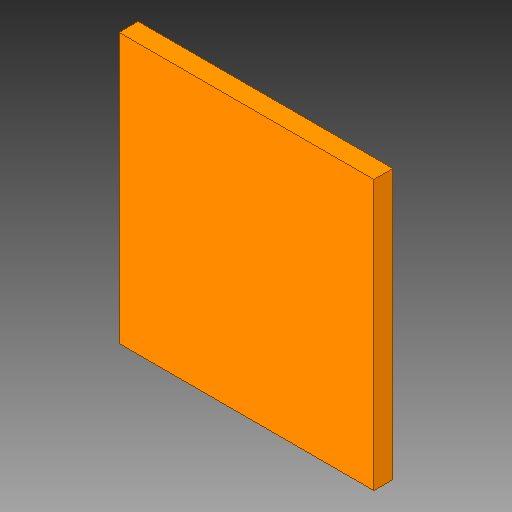
# Autodesk Inventor part: MSP430F5529IPNR
Saved by Autodesk Inventor 2018 (Build 220112000, 112)
## iProperties
Created: 2015-11-24
Part Number: MSP430F5529IPNR
Material: Generic
Document SubType Name: Modeling
Designer: PhillipD
Density: 1 g/cm^3
Appearance: PN80, MSP430F5529IPNR
Author: PhillipD
Autodesk Inventor part; units mm, degrees
ref_plane "YZ Plane" through (0, 0, 0) normal (1, 0, 0) x (0, 1, 0)
ref_plane "XZ Plane" through (0, 0, 0) normal (0, 1, 0) x (-1, 0, 0)
ref_plane "XY Plane" through (0, 0, 0) normal (0, 0, 1) x (1, 0, 0)
sketch "PN80, MSP430F5529IPNR_171" plane through (0, 0, 0) normal (0, 0, 1) x (1, 0, 0)
  line L0 (-6.71, 7.095) -> (6.71, 7.095)
  line L1 (6.71, 7.095) -> (6.71, -7.095)
  line L2 (6.71, -7.095) -> (-6.71, -7.095)
  line L3 (-6.71, -7.095) -> (-6.71, 7.095)
  constraints: 8 end point
extrude "Extrusion1" add sketch "PN80, MSP430F5529IPNR_171" along normal blind 1
body "Solid1"
